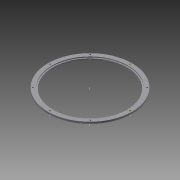
# Autodesk Inventor part: Shield Support Ring
Saved by Autodesk Inventor 2015 (Build 190159000, 159)
## iProperties
Created: 2014-07-02
Part Number: Shield Support Ring
Material: Generic
Document SubType Name: Modeling
Designer: Aki
Density: 1 g/cm^3
Appearance: Default
Author: Aki
Autodesk Inventor part; units mm, degrees
ref_plane "YZ Plane" through (0, 0, 0) normal (1, 0, 0) x (0, 1, 0)
ref_plane "XZ Plane" through (0, 0, 0) normal (0, 1, 0) x (-1, 0, 0)
ref_plane "XY Plane" through (0, 0, 0) normal (0, 0, 1) x (1, 0, 0)
sketch "Sketch1" plane through (0, 0, 0) normal (0, 1, 0) x (-1, 0, 0)
  circle A0 centre (0, 0) radius 94
  dimension "d0" = 188
  constraints: 1 centre point, 1 coincident
  measures "d0" diameter of A0
extrude "Extrusion1" add sketch "Sketch1" along normal blind 4
sketch "Sketch2" plane through (0, 4, 0) normal (0, 1, 0) x (1, 0, 0)
  circle A0 centre (0, 0) radius 87.5
  dimension "d3" = 175
  constraints: 1 centre point, 1 coincident
  measures "d3" diameter of A0
hole "Hole1" at (0, 4, 0) direction (0, -1, 0) diameter 170 depth 2
sketch "Sketch3" plane through (0, 2, 0) normal (0, 1, 0) x (1, 0, 0)
  circle A0 centre (0, 0) radius 82
  dimension "d11" = 164
  constraints: 1 centre point, 1 coincident
  measures "d11" diameter of A0
hole "Hole2" at (0, 2, 0) direction (0, -1, 0) diameter 165 end through all
sketch "Sketch4" plane through (0, 4, 0) normal (0, 1, 0) x (1, 0, 0)
  circle A0 centre (-90, 0) radius 1.65
  point P0 (0, 0)
  dimension "d19" = 3.3
  dimension "d20" = 90
  constraints: 1 centre point
  measures "d19" diameter of A0
  measures "d20" distance of point (0, 0) A0.centre
sketch "Sketch5" plane through (0, 4, 0) normal (0, 1, 0) x (1, 0, 0)
  circle A0 centre (-63.6396, 63.6396) radius 1.65
  point P0 (0, 0)
  dimension "d28" = 3.3
  dimension "d29" = 90
  dimension "d33" = 63.6396
  constraints: 1 centre point
  measures "d28" diameter of A0
  measures "d29" distance of point (0, 0) A0.centre
  measures "d33" horizontal distance of point (0, 0) A0.centre
sketch "Sketch6" plane through (0, 4, 0) normal (0, 1, 0) x (1, 0, 0)
  circle A0 centre (0, 90) radius 1.65
  point P0 (0, 0)
  dimension "d34" = 3.3
  dimension "d35" = 90
  constraints: 1 centre point
  measures "d34" diameter of A0
  measures "d35" distance of point (0, 0) A0.centre
sketch "Sketch7" plane through (0, 4, 0) normal (0, 1, 0) x (1, 0, 0)
  circle A0 centre (63.6396, 63.6396) radius 1.65
  point P0 (0, 0)
  dimension "d36" = 3.3
  dimension "d37" = 90
  dimension "d38" = 63.6396
  dimension "d121" = 63.6396
  constraints: 1 centre point
  measures "d36" diameter of A0
  measures "d37" distance of point (0, 0) A0.centre
  measures "d38" horizontal distance of point (0, 0) A0.centre
  measures "d121" horizontal distance of point (0, 0) A0.centre
sketch "Sketch8" plane through (0, 4, 0) normal (0, 1, 0) x (1, 0, 0)
  circle A0 centre (90, 0) radius 1.65
  point P0 (0, 0)
  dimension "d39" = 3.3
  dimension "d40" = 90
  constraints: 1 centre point
  measures "d39" diameter of A0
  measures "d40" distance of A0.centre point (0, 0)
sketch "Sketch9" plane through (0, 4, 0) normal (0, 1, 0) x (1, 0, 0)
  circle A0 centre (63.6396, -63.6396) radius 2.15
  point P0 (0, 0)
  dimension "d41" = 4.3
  dimension "d42" = 90
  dimension "d43" = 63.6396
  dimension "d122" = 63.6396
  constraints: 1 centre point
  measures "d41" diameter of A0
  measures "d42" distance of A0.centre point (0, 0)
  measures "d43" horizontal distance of point (0, 0) A0.centre
  measures "d122" horizontal distance of point (0, 0) A0.centre
sketch "Sketch10" plane through (0, 4, 0) normal (0, 1, 0) x (1, 0, 0)
  circle A0 centre (0, -90) radius 1.65
  point P0 (0, 0)
  dimension "d44" = 3.3
  dimension "d45" = 90
  constraints: 1 centre point
  measures "d44" diameter of A0
  measures "d45" distance of A0.centre point (0, 0)
sketch "Sketch11" plane through (0, 4, 0) normal (0, 1, 0) x (1, 0, 0)
  circle A0 centre (-63.6396, -63.6396) radius 1.65
  point P0 (0, 0)
  dimension "d46" = 3.3
  dimension "d47" = 90
  dimension "d48" = 63.6396
  dimension "d123" = 63.6396
  constraints: 1 centre point
  measures "d46" diameter of A0
  measures "d47" distance of point (0, 0) A0.centre
  measures "d48" horizontal distance of point (0, 0) A0.centre
  measures "d123" horizontal distance of point (0, 0) A0.centre
hole "Hole4" at (-90, 4, 0) direction (0, -1, 0) diameter 3.3 end through all
hole "Hole5" at (-63.6396, 4, -63.6396) direction (0, -1, 0) diameter 3.3 end through all
hole "Hole6" at (0, 4, -90) direction (0, -1, 0) diameter 3.3 end through all
hole "Hole7" at (63.6396, 4, -63.6396) direction (0, -1, 0) diameter 3.3 end through all
hole "Hole8" at (90, 4, 0) direction (0, -1, 0) diameter 3.3 end through all
hole "Hole9" at (63.6396, 4, 63.6396) direction (0, -1, 0) diameter 3.3 end through all
hole "Hole10" at (0, 4, 90) direction (0, -1, 0) diameter 3.3 end through all
hole "Hole11" at (-63.6396, 4, 63.6396) direction (0, -1, 0) diameter 3.3 end through all
thread "Thread9" size "M3.5x0.6" class "6H" standard "ANSI Metric M Profile" full length
thread "Thread10" size "M3.5x0.6" class "6H" standard "ANSI Metric M Profile" full length
thread "Thread11" size "M3.5x0.6" class "6H" standard "ANSI Metric M Profile" full length
thread "Thread12" size "M3.5x0.6" class "6H" standard "ANSI Metric M Profile" full length
thread "Thread13" size "M3.5x0.6" class "6H" standard "ANSI Metric M Profile" full length
thread "Thread14" size "M3.5x0.6" class "6H" standard "ANSI Metric M Profile" full length
thread "Thread15" size "M3.5x0.6" class "6H" standard "ANSI Metric M Profile" full length
thread "Thread16" size "M3.5x0.6" class "6H" standard "ANSI Metric M Profile" full length
thread "Thread17" size "M3.5x0.6" class "6H" standard "ANSI Metric M Profile" full length
body "Solid1"
